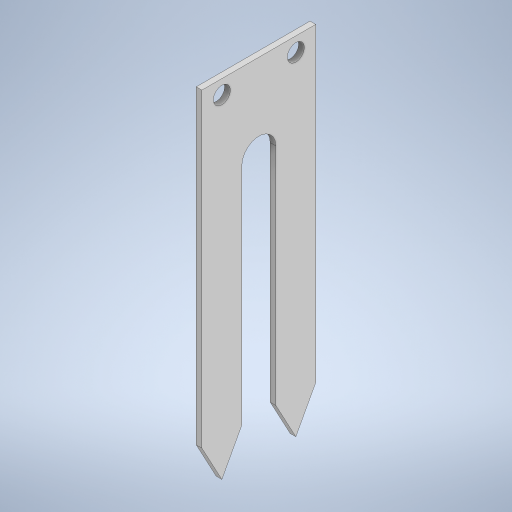
# Autodesk Inventor part: moisture sensor
Saved by Autodesk Inventor 2023 (Build 270158000, 158)
## iProperties
Created: 2023-04-03
Part Number: moisture sensor
Material: Generic
Document SubType Name: Modeling
Designer: user
Density: 1 g/cm^3
Appearance: Default
Author: user
Autodesk Inventor part; units mm, degrees
ref_plane "YZ Plane" through (0, 0, 0) normal (1, 0, 0) x (0, 1, 0)
ref_plane "XZ Plane" through (0, 0, 0) normal (0, 1, 0) x (-1, 0, 0)
ref_plane "XY Plane" through (0, 0, 0) normal (0, 0, 1) x (1, 0, 0)
sketch "Sketch1" plane through (0, 0, 0) normal (1, 0, 0) x (0, 1, 0)
  line L0 (1.3538, 1) -> (1.3538, -1)
  line L1 (1.3538, -1) -> (-4.0962, -1)
  line L2 (-4.0962, -1) -> (-4.7462, -0.65)
  line L3 (-4.7462, -0.65) -> (-4.0962, -0.3)
  line L4 (-4.0962, -0.3) -> (-0.1462, -0.3)
  line L5 (-0.1462, 0.3) -> (-4.0962, 0.3)
  line L6 (-4.0962, 0.3) -> (-4.7462, 0.65)
  line L7 (-4.7462, 0.65) -> (-4.0962, 1)
  line L8 (-4.0962, 1) -> (1.3538, 1)
  arc A0 (-0.1462, -0.3) -> (-0.1462, 0.3) centre (-0.1462, 0) ccw
  circle A1 centre (1.1038, 0.65) radius 0.15
  circle A2 centre (1.1038, -0.65) radius 0.15
  point P0 (0, 0)
  point P1 (-1.3712, -1)
  dimension "d0" = 2
  dimension "d1" = 5.45
  dimension "d2" = 0.7
  dimension "d3" = 0.7
  dimension "d4" = 0.65
  dimension "d6" = 1.3538
  dimension "d7" = 3.95
  dimension "d8" = 3.95
  dimension "d9" = 0.3
  dimension "d10" = 0.6
  dimension "d11" = 1
  dimension "d12" = 6.1
  dimension "d13" = 0.1462
  dimension "d14" = 5.45
  dimension "d16" = 0.3
  dimension "d17" = 0.35
  dimension "d19" = 0.1
  dimension "d20" = 0.1
  dimension "d21" = 0.35
  dimension "d22" = 0.35
  dimension "d23" = 0.65
  dimension "d24" = 0.65
  dimension "d25" = 0.35
  dimension "d26" = 0.35
  dimension "d27" = 0.65
  dimension "d28" = 0.3
  dimension "d31" = 0.65
  constraints: 18 end point, 3 centre point, 2 horizontal, 2 point on circle, 1 midpoint, 1 parallel, 1 vertical
  measures "d0" distance of L0.start L0.end
  measures "d1" distance of L0.end L1.end
  measures "d2" distance from line of L4 point (-1.371, -1)
  measures "d3" distance between parallel lines of L8 L5
  measures "d4" horizontal distance of L1.end L2.end
  measures "d6" distance from line of point (0, 0) L0
  measures "d7" distance of L3.end L4.end
  measures "d8" distance of L5.start L5.end
  measures "d9" radius of A0
  measures "d10" distance between parallel lines of L5 L4
  measures "d11" distance from line of L1 point (0, 0)
  measures "d12" distance from line of L2.end L0
  measures "d13" distance of point (0, 0) A0.centre
  measures "d14" distance of L7.end L8.end
  measures "d16" diameter of A2
  measures "d17" distance from line of L8 A1.centre
  measures "d19" distance edge to line of A1 L0
  measures "d20" distance edge to line of A2 L0
  measures "d21" vertical distance of L1.end L2.end
  measures "d22" vertical distance of L2.end L3.end
  measures "d23" horizontal distance of L3.end L2.end
  measures "d24" horizontal distance of L6.end L5.end
  measures "d25" vertical distance of L6.end L5.end
  measures "d26" vertical distance of L7.end L6.end
  measures "d27" horizontal distance of L7.end L6.end
  measures "d28" diameter of A1
  measures "d31" vertical distance of point (0, 0) A2.centre
extrude "Extrusion1" add sketch "Sketch1" along normal blind 0.1
equation "\"d14\" = d1"
body "Solid1"
